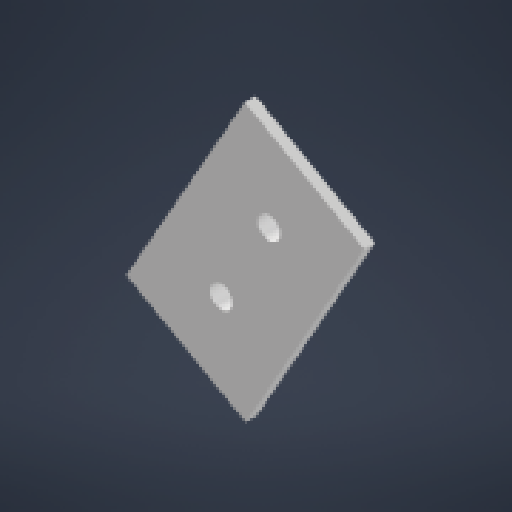
# Autodesk Inventor part: Bottom_Claw_Mount
Saved by Autodesk Inventor 2024.2 (Build 282272000, 272)
## iProperties
Created: 2024-06-18
Part Number: Bottom_Claw_Mount
Material: Generic
Document SubType Name: Modeling
Designer: warm
Density: 1 g/cm^3
Appearance: Default
Author: warm
Autodesk Inventor part; units mm, degrees
ref_plane "YZ Plane" through (0, 0, 0) normal (1, 0, 0) x (0, 1, 0)
ref_plane "XZ Plane" through (0, 0, 0) normal (0, 1, 0) x (-1, 0, 0)
ref_plane "XY Plane" through (0, 0, 0) normal (0, 0, 1) x (1, 0, 0)
sketch "Sketch1" plane through (0, 0, 0) normal (0, 0, 1) x (1, 0, 0)
  circle A0 centre (0, 0) radius 6.4
  circle A1 centre (0, 0) radius 4.73
  circle A2 centre (0, 0) radius 4.15
  circle A3 centre (0, 0) radius 7.3
  point P0 (0, 0)
  constraints: 4 centre point, 8 other
extrude "Extrusion1" add sketch "Sketch1" along normal blind 4 contours A1
ref_plane "Work Plane1" through (17.5111, 30.8959, 0) normal (0, 0, 1) x (1, 0, 0)
sketch "Sketch2" plane through (17.5111, 30.8959, 0) normal (0, 0, 1) x (1, 0, 0)
  circle A0 centre (0, 0) radius 6.4
  circle A1 centre (0, 0) radius 4.73
  circle A2 centre (0, 0) radius 4.15
  circle A3 centre (0, 0) radius 7.3
  point P0 (-17.5111, -30.8959)
  constraints: 4 centre point, 8 other
extrude "Extrusion2" add sketch "Sketch2" along normal blind 4 contours A1
sketch "Sketch3" plane through (17.5111, 30.8959, 4) normal (0, 0, 1) x (1, 0, 0)
  circle A0 centre (-17.5111, -30.8959) radius 4.15 projected
  circle A1 centre (-17.5111, -30.8959) radius 4.73 projected
  circle A2 centre (0, 0) radius 4.15 projected
  circle A3 centre (0, 0) radius 4.73 projected
  line L0 (0, 0) -> (-17.5111, -30.8959) construction
  line L1 (-52.7707, -41.5942) -> (-8.9354, 35.7471)
  line L2 (-8.9354, 35.7471) -> (35.2596, 10.6983)
  line L3 (35.2596, 10.6983) -> (-8.5757, -66.643)
  line L4 (-8.5757, -66.643) -> (-52.7707, -41.5942)
  line L5 (-52.7707, -41.5942) -> (35.2596, 10.6983) construction
  line L6 (-8.9354, 35.7471) -> (-8.5757, -66.643) construction
  point P0 (-17.5111, -30.8959)
  point P1 (-8.7555, -15.448)
  dimension "d4" = 88.9
  dimension "d5" = 50.8
  constraints: 14 end point, 3 midpoint, 3 parallel, 1 perpendicular
  measures "d4" distance of L1.start L1.end
  measures "d5" distance of L1.end L2.end
extrude "Extrusion3" add sketch "Sketch3" along normal blind 4 contours A1 | A3 | L1 L2 L3 L4
fillet "Fillet1" radius 3.175 1 edges at (12.7811, 30.8959, 4)
fillet "Fillet2" radius 3.175 1 edges at (-4.73, 0, 4)
sketch "Sketch4" plane through (17.5111, 30.8959, 8) normal (0, 0, 1) x (1, 0, 0)
  line L0 (-8.5757, -66.643) -> (-52.7707, -41.5942) projected
  line L1 (-52.7707, -41.5942) -> (-8.9354, 35.7471) projected
  line L2 (-8.9354, 35.7471) -> (35.2596, 10.6983) projected
  line L3 (35.2596, 10.6983) -> (-8.5757, -66.643) projected
  circle A0 centre (-17.5111, -30.8959) radius 4.15 projected
  circle A1 centre (0, 0) radius 4.15 projected
  circle A2 centre (0, 0) radius 4 projected
  circle A3 centre (-17.5111, -30.8959) radius 4 projected
  point P0 (-17.5111, -30.8959)
extrude "Extrusion4" add sketch "Sketch4" against normal blind 30.1388 contours A2
fillet "Fillet3" radius 0.3969 1 edges at (13.5111, 30.8959, -22.1388)
sketch "Sketch5" plane through (17.5111, 30.8959, 8) normal (0, 0, 1) x (1, 0, 0)
  circle A0 centre (-17.5111, -30.8959) radius 4 projected
  point P0 (-17.5111, -30.8959)
extrude "Extrusion5" add sketch "Sketch5" against normal blind 12.065
sketch "Sketch6" plane through (17.5111, 30.8959, 8) normal (0, 0, 1) x (1, 0, 0)
  line L0 (-8.5757, -66.643) -> (35.2596, 10.6983) projected
  line L1 (35.2596, 10.6983) -> (-8.9354, 35.7471) projected
  line L2 (-8.9354, 35.7471) -> (-52.7707, -41.5942) projected
  line L3 (-52.7707, -41.5942) -> (-8.5757, -66.643) projected
  circle A0 centre (-17.5111, -30.8959) radius 4.15 projected
  circle A1 centre (0, 0) radius 4.15 projected
  point P0 (-17.5111, -30.8959)
extrude "Extrusion6" add sketch "Sketch6" against normal blind 6.985 contours A0 | A1
sketch "Sketch8" plane through (0, 0, -4.065) normal (0, 0, -1) x (-1, 0, 0)
  circle A0 centre (0, 0) radius 4 projected
  circle A1 centre (0, 0) radius 2
  point P0 (0, 0)
  dimension "d20" = 4
  constraints: 1 centre point, 1 coincident
  measures "d20" diameter of A1
extrude "Extrusion8" cut sketch "Sketch8" against normal blind 8 contours A1
fillet "Fillet4" radius 0.3969 1 edges at (-4, 0, -4.065)
ref_plane "Work Plane2" through (17.5111, 30.8959, -12.7) normal (0, 0, -1) x (-0.8699899, 0.4930696, 0)
sketch "Sketch7" plane through (17.5111, 30.8959, -22.1388) normal (0, 0, -1) x (-1, 0, 0)
  circle A0 centre (0, 0) radius 3.6031 projected
  circle A1 centre (0, 0) radius 1.9
  point P0 (17.5111, -30.8959)
  dimension "d17" = 3.8
  constraints: 1 centre point, 1 coincident
  measures "d17" diameter of A1
extrude "Extrusion7" cut sketch "Sketch7" against normal blind 8 contours A1
sketch "Sketch9" plane through (17.5111, 30.8959, -12.7) normal (0, 0, -1) x (-0.8699899, 0.4930696, 0)
  circle A0 centre (0, 0) radius 6.4
  circle A1 centre (0, 0) radius 4.73
  circle A2 centre (0, 0) radius 4.15
  circle A3 centre (0, 0) radius 7.3
  circle A4 centre (0, 0) radius 1.9 projected
  point P0 (0.0006, -35.5133)
  constraints: 4 centre point, 8 other
extrude "Extrusion9" add sketch "Sketch9" along normal blind 0.5 contours A1 | A2 | A4
fillet "Fillet5" radius 3.175 1 edges at (13.5111, 30.8959, -13.2)
body "Solid1"
